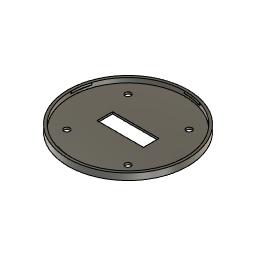
Thermostat Assembly_ (Autodesk Fusion 360 archive; units mm, degrees)
design "Thermostat Base"
Autodesk Fusion 360 part; units mm, degrees
sketch "Sketch1" plane through (0, 0, 0) normal (0, 0, 1) x (1, 0, 0)
cylinder "CylinderPrimitive1" add diameter 98.2472 height 1.5875 placed x (1, 0, 0) y (0, 1, 0) z (0, 0, 1) at (0, 0, 0)
sketch "Sketch3" plane through (0, 0, 1.5875) normal (0, 0, 1) x (-1, 0, 0)
  circle A0 centre (0, 0) radius 49.1236
  line L0 (-19.05, 6.35) -> (19.05, 6.35)
  line L1 (19.05, 6.35) -> (19.05, -6.35)
  line L2 (19.05, -6.35) -> (-19.05, -6.35)
  line L3 (-19.05, -6.35) -> (-19.05, 6.35)
  line L4 (-19.05, 6.35) -> (19.05, -6.35) construction
  line L5 (19.05, 6.35) -> (-19.05, -6.35) construction
  dimension "d3" = 38.1
  dimension "d4" = 12.7
  constraint horizontal L0
  constraint perpendicular L0 L1
  constraint parallel L0 L2
  constraint parallel L1 L3
  constraint coincident L4 A0.centre
  constraint coincident L5 A0.centre
  constraint coincident A0.centre origin
  measures "d3" distance of L1.end L2.end
  measures "d4" distance of L0.end L1.end
extrude "Extrude1" cut sketch "Sketch3" against normal blind 54.4068 contours L0 L1 L2 L3
sketch "Sketch4" plane through (0, 0, 1.5875) normal (0, 0, 1) x (-1, 0, 0)
  line L0 (19.05, 6.35) -> (19.05, -6.35)
  line L1 (19.05, -6.35) -> (-19.05, -6.35)
  line L2 (-19.05, -6.35) -> (-19.05, 6.35)
  line L3 (-19.05, 6.35) -> (19.05, 6.35)
  circle A0 centre (0, 0) radius 49.1236
  line L4 (0, 0) -> (31.75, 0) construction
  line L5 (0, 0) -> (25.1447, -25.1447)
  line L6 (0, 0) -> (35.56, 0) construction
  line L7 (0, 0) -> (-25.1447, -25.1447)
  line L8 (0, 0) -> (35.56, 0) construction
  line L9 (0, 0) -> (25.1447, 25.1447)
  line L10 (0, 0) -> (-25.1447, 25.1447)
  line L11 (0, 0) -> (-35.56, 0) construction
  circle A1 centre (25.1447, -25.1447) radius 2.413
  circle A2 centre (-25.1447, -25.1447) radius 2.413
  circle A3 centre (25.1447, 25.1447) radius 2.413
  circle A4 centre (-25.1447, 25.1447) radius 2.413
  dimension "d14" = 45
  dimension "d15" = 35.56
  dimension "d16" = 135
  dimension "d17" = 35.56
  dimension "d18" = 35.56
  dimension "d19" = 45
  dimension "d20" = 35.56
  dimension "d21" = 4.826
  dimension "d22" = 4.826
  dimension "d23" = 4.826
  dimension "d24" = 4.826
  constraint coincident A0.centre L4.start
  constraint horizontal L4
  constraint horizontal L6
  constraint horizontal L8
  constraint perpendicular L5 L9
  constraint horizontal L11
  constraint coincident L5.end A1.centre
  constraint coincident L7.end A2.centre
  constraint coincident L9.end A3.centre
  constraint coincident L10.end A4.centre
  measures "d14" angle of L5 L6
  measures "d15" distance of A0.centre L5.end
  measures "d16" angle of L7 L8
  measures "d17" distance of A0.centre L7.end
  measures "d18" distance of A0.centre L9.end
  measures "d19" angle of L10 L11
  measures "d20" distance of A0.centre L10.end
  measures "d21" diameter of A1
  measures "d22" diameter of A2
  measures "d23" diameter of A3
  measures "d24" diameter of A4
extrude "Extrude2" cut sketch "Sketch4" against normal blind 18.9738 contours A1 | A2 | A3 | A4
sketch "Sketch5" plane through (0, 0, 0) normal (0, 0, 1) x (1, 0, 0)
cylinder "CylinderPrimitive2" add diameter 98.2472 height 3.81 placed x (1, 0, 0) y (0, 1, 0) z (0, 0, 1) at (0, 0, 1.5875)
hole "Hole1" at (0, 0, 5.3975) direction (0, 0, -1) diameter 93.98 depth 3.81 tip angle 180
sketch "Sketch14" plane through (0, 0, 0) normal (0, 1, 0) x (1, 0, 0)
  line L0 (46.99, -5.3975) -> (-46.99, -5.3975)
  line L1 (-46.99, -5.3975) -> (-46.99, -3.4925)
  line L2 (-46.99, -3.4925) -> (-46.0375, -4.445)
  line L3 (-46.0375, -4.445) -> (-46.99, -5.3975)
  line L4 (-46.0375, -4.445) -> (-46.99, -4.445) construction
  dimension "d39" = 1.905
  dimension "d40" = 0.9525
  constraint coincident L0.end L1.start
  constraint perpendicular L0 L1
  constraint equal L2 L3
  constraint midpoint L1 L4.end
  measures "d39" distance of L0.end L1.end
  measures "d40" distance of L2.end L4.end
revolve "Revolve2" add sketch "Sketch14" angle 18 about axis through (0, 0, 5.3975) along (0, 0, -1)
pattern_circular "C-Pattern1" count 4 over 360 about axis through (0, 0, 5.3975) along (0, 0, -1) of "Revolve2"
equation "d2 = 3.7 in + 0.168 in"
equation "d28 = 3.70 in + 0.168 in"

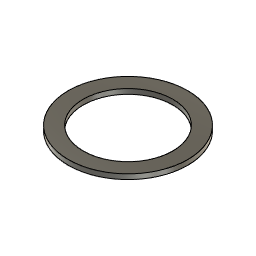
design "IR Sensor Shield/Bearing"
Autodesk Fusion 360 part; units mm, degrees
cylinder "CylinderPrimitive1" add diameter 19.05 height 0.7937 placed x (1, 0, 0) y (0, 1, 0) z (0, 0, 1) at (0, 0, 0)
hole "Hole1" at (0, 0, 0.7937) direction (0, 0, -1) diameter 14.3002 depth 7.62 tip angle 180
equation "d1 = ( 0.5 / 16 ) * 1 in"
